Autodesk Inventor part; units mm, degrees
(part 2 of 2)
sketch "Náčrt2 outline for Vysunutí2" plane through (-3.809999, 5.08, 0) normal (0, 1, 0) x (1, 0, 0)
  line L0 (-2.971901, 1.32351) -> (-1.677758, 1.064456)
  line L1 (-2.990322, 1.327194) -> (-2.971901, 1.32351)
  arc A0 (-3.389, 1.845748) -> (-2.990322, 1.327194) centre (-2.881505, 1.82339) ccw
  line L2 (-3.389, 2.240304) -> (-3.389, 1.845748)
  arc A1 (-2.97646, 2.739034) -> (-3.389, 2.240304) centre (-2.881172, 2.240226) ccw
  line L3 (-1.678461, 2.998415) -> (-2.97646, 2.739034)
  arc A2 (-1.27, 3.497336) -> (-1.678461, 2.998415) centre (-1.778009, 3.496575) cw
  line L4 (-1.27, 0.566986) -> (-1.27, 3.497336)
  arc A3 (-1.677758, 1.064456) -> (-1.27, 0.566986) centre (-1.777338, 0.566986) cw
  line L5 (-2.971901, 87.172837) -> (-1.677758, 86.913783)
  line L6 (-2.990322, 87.176521) -> (-2.971901, 87.172837)
  arc A4 (-3.389, 87.695075) -> (-2.990322, 87.176521) centre (-2.881505, 87.672717) ccw
  line L7 (-3.389, 88.089631) -> (-3.389, 87.695075)
  arc A5 (-2.97646, 88.588361) -> (-3.389, 88.089631) centre (-2.881172, 88.089553) ccw
  line L8 (-1.678461, 88.847742) -> (-2.97646, 88.588361)
  arc A6 (-1.27, 89.346664) -> (-1.678461, 88.847742) centre (-1.778009, 89.345902) cw
  line L9 (-1.27, 86.416314) -> (-1.27, 89.346664)
  arc A7 (-1.677758, 86.913783) -> (-1.27, 86.416314) centre (-1.777338, 86.416314) cw
  line L10 (-2.971901, 83.87094) -> (-1.677758, 83.611886)
  line L11 (-2.990322, 83.874624) -> (-2.971901, 83.87094)
  arc A8 (-3.389, 84.393178) -> (-2.990322, 83.874624) centre (-2.881505, 84.37082) ccw
  line L12 (-3.389, 84.78802) -> (-3.389, 84.393178)
  arc A9 (-2.97646, 85.286464) -> (-3.389, 84.78802) centre (-2.881172, 84.787656) ccw
  line L13 (-1.678461, 85.545844) -> (-2.97646, 85.286464)
  arc A10 (-1.27, 86.044766) -> (-1.678461, 85.545844) centre (-1.778009, 86.044005) cw
  line L14 (-1.27, 83.114416) -> (-1.27, 86.044766)
  arc A11 (-1.677758, 83.611886) -> (-1.27, 83.114416) centre (-1.777338, 83.114416) cw
  line L15 (-2.971901, 80.569043) -> (-1.677758, 80.309989)
  line L16 (-2.990322, 80.572727) -> (-2.971901, 80.569043)
  arc A12 (-3.389, 81.091281) -> (-2.990322, 80.572727) centre (-2.881505, 81.068923) ccw
  line L17 (-3.389, 81.486123) -> (-3.389, 81.091281)
  arc A13 (-2.97646, 81.984567) -> (-3.389, 81.486123) centre (-2.881172, 81.485759) ccw
  line L18 (-1.678461, 82.243947) -> (-2.97646, 81.984567)
  arc A14 (-1.27, 82.742869) -> (-1.678461, 82.243947) centre (-1.778009, 82.742108) cw
  line L19 (-1.27, 79.812519) -> (-1.27, 82.742869)
  arc A15 (-1.677758, 80.309989) -> (-1.27, 79.812519) centre (-1.777338, 79.812519) cw
  line L20 (-2.971901, 77.267146) -> (-1.677758, 77.008092)
  line L21 (-2.990322, 77.27083) -> (-2.971901, 77.267146)
  arc A16 (-3.389, 77.789383) -> (-2.990322, 77.27083) centre (-2.881505, 77.767025) ccw
  line L22 (-3.389, 78.184226) -> (-3.389, 77.789383)
  arc A17 (-2.97646, 78.68267) -> (-3.389, 78.184226) centre (-2.881172, 78.183862) ccw
  line L23 (-1.678461, 78.94205) -> (-2.97646, 78.68267)
  arc A18 (-1.27, 79.440972) -> (-1.678461, 78.94205) centre (-1.778009, 79.440211) cw
  line L24 (-1.27, 76.510622) -> (-1.27, 79.440972)
  arc A19 (-1.677758, 77.008092) -> (-1.27, 76.510622) centre (-1.777338, 76.510622) cw
  line L25 (-2.971901, 73.965248) -> (-1.677758, 73.706195)
  line L26 (-2.990322, 73.968933) -> (-2.971901, 73.965248)
  arc A20 (-3.389, 74.487486) -> (-2.990322, 73.968933) centre (-2.881505, 74.465128) ccw
  line L27 (-3.389, 74.882329) -> (-3.389, 74.487486)
  arc A21 (-2.97646, 75.380772) -> (-3.389, 74.882329) centre (-2.881172, 74.881964) ccw
  line L28 (-1.678461, 75.640153) -> (-2.97646, 75.380772)
  arc A22 (-1.27, 76.139075) -> (-1.678461, 75.640153) centre (-1.778009, 76.138314) cw
  line L29 (-1.27, 73.208725) -> (-1.27, 76.139075)
  arc A23 (-1.677758, 73.706195) -> (-1.27, 73.208725) centre (-1.777338, 73.208725) cw
  line L30 (-2.971901, 70.663351) -> (-1.677758, 70.404297)
  line L31 (-2.990322, 70.667035) -> (-2.971901, 70.663351)
  arc A24 (-3.389, 71.185589) -> (-2.990322, 70.667035) centre (-2.881505, 71.163231) ccw
  line L32 (-3.389, 71.580145) -> (-3.389, 71.185589)
  arc A25 (-2.97646, 72.078875) -> (-3.389, 71.580145) centre (-2.881172, 71.580067) ccw
  line L33 (-1.678461, 72.338256) -> (-2.97646, 72.078875)
  arc A26 (-1.27, 72.837178) -> (-1.678461, 72.338256) centre (-1.778009, 72.836416) cw
  line L34 (-1.27, 69.906828) -> (-1.27, 72.837178)
  arc A27 (-1.677758, 70.404297) -> (-1.27, 69.906828) centre (-1.777338, 69.906828) cw
  line L35 (-2.971901, 67.361454) -> (-1.677758, 67.1024)
  line L36 (-2.990322, 67.365138) -> (-2.971901, 67.361454)
  arc A28 (-3.389, 67.883692) -> (-2.990322, 67.365138) centre (-2.881505, 67.861334) ccw
  line L37 (-3.389, 68.278534) -> (-3.389, 67.883692)
  arc A29 (-2.97646, 68.776978) -> (-3.389, 68.278534) centre (-2.881172, 68.27817) ccw
  line L38 (-1.678461, 69.036358) -> (-2.97646, 68.776978)
  arc A30 (-1.27, 69.53528) -> (-1.678461, 69.036358) centre (-1.778009, 69.534519) cw
  line L39 (-1.27, 66.60493) -> (-1.27, 69.53528)
  arc A31 (-1.677758, 67.1024) -> (-1.27, 66.60493) centre (-1.777338, 66.60493) cw
  line L40 (-2.971901, 64.059557) -> (-1.677758, 63.800503)
  line L41 (-2.990322, 64.063241) -> (-2.971901, 64.059557)
  arc A32 (-3.389, 64.581795) -> (-2.990322, 64.063241) centre (-2.881505, 64.559437) ccw
  line L42 (-3.389, 64.976351) -> (-3.389, 64.581795)
  arc A33 (-2.97646, 65.475081) -> (-3.389, 64.976351) centre (-2.881172, 64.976273) ccw
  line L43 (-1.678461, 65.734461) -> (-2.97646, 65.475081)
  arc A34 (-1.27, 66.233383) -> (-1.678461, 65.734461) centre (-1.778009, 66.232622) cw
  line L44 (-1.27, 63.303033) -> (-1.27, 66.233383)
  arc A35 (-1.677758, 63.800503) -> (-1.27, 63.303033) centre (-1.777338, 63.303033) cw
  line L45 (-2.971901, 60.75766) -> (-1.677758, 60.498606)
  line L46 (-2.990322, 60.761344) -> (-2.971901, 60.75766)
  arc A36 (-3.389, 61.279897) -> (-2.990322, 60.761344) centre (-2.881505, 61.257539) ccw
  line L47 (-3.389, 61.67474) -> (-3.389, 61.279897)
  arc A37 (-2.97646, 62.173184) -> (-3.389, 61.67474) centre (-2.881172, 61.674376) ccw
  line L48 (-1.678461, 62.432564) -> (-2.97646, 62.173184)
  arc A38 (-1.27, 62.931486) -> (-1.678461, 62.432564) centre (-1.778009, 62.930725) cw
  line L49 (-1.27, 60.001136) -> (-1.27, 62.931486)
  arc A39 (-1.677758, 60.498606) -> (-1.27, 60.001136) centre (-1.777338, 60.001136) cw
  line L50 (-2.971901, 57.455762) -> (-1.677758, 57.196709)
  line L51 (-2.990322, 57.459447) -> (-2.971901, 57.455762)
  arc A40 (-3.389, 57.978) -> (-2.990322, 57.459447) centre (-2.881505, 57.955642) ccw
  line L52 (-3.389, 58.372843) -> (-3.389, 57.978)
  arc A41 (-2.97646, 58.871286) -> (-3.389, 58.372843) centre (-2.881172, 58.372478) ccw
  line L53 (-1.678461, 59.130667) -> (-2.97646, 58.871286)
  arc A42 (-1.27, 59.629589) -> (-1.678461, 59.130667) centre (-1.778009, 59.628828) cw
  line L54 (-1.27, 56.699239) -> (-1.27, 59.629589)
  arc A43 (-1.677758, 57.196709) -> (-1.27, 56.699239) centre (-1.777338, 56.699239) cw
  line L55 (-2.971901, 54.153865) -> (-1.677758, 53.894811)
  line L56 (-2.990322, 54.15755) -> (-2.971901, 54.153865)
  arc A44 (-3.389, 54.676103) -> (-2.990322, 54.15755) centre (-2.881505, 54.653745) ccw
  line L57 (-3.389, 55.070946) -> (-3.389, 54.676103)
  arc A45 (-2.97646, 55.569389) -> (-3.389, 55.070946) centre (-2.881172, 55.070581) ccw
  line L58 (-1.678461, 55.82877) -> (-2.97646, 55.569389)
  arc A46 (-1.27, 56.327692) -> (-1.678461, 55.82877) centre (-1.778009, 56.32693) cw
  line L59 (-1.27, 53.397342) -> (-1.27, 56.327692)
  arc A47 (-1.677758, 53.894811) -> (-1.27, 53.397342) centre (-1.777338, 53.397342) cw
  line L60 (-2.971901, 50.851968) -> (-1.677758, 50.592914)
  line L61 (-2.990322, 50.855652) -> (-2.971901, 50.851968)
  arc A48 (-3.389, 51.374206) -> (-2.990322, 50.855652) centre (-2.881505, 51.351848) ccw
  line L62 (-3.389, 51.769048) -> (-3.389, 51.374206)
  arc A49 (-2.97646, 52.267492) -> (-3.389, 51.769048) centre (-2.881172, 51.768684) ccw
  line L63 (-1.678461, 52.526873) -> (-2.97646, 52.267492)
  arc A50 (-1.27, 53.025794) -> (-1.678461, 52.526873) centre (-1.778009, 53.025033) cw
  line L64 (-1.27, 50.095444) -> (-1.27, 53.025794)
  arc A51 (-1.677758, 50.592914) -> (-1.27, 50.095444) centre (-1.777338, 50.095444) cw
  line L65 (-2.971901, 47.550071) -> (-1.677758, 47.291017)
  line L66 (-2.990322, 47.553755) -> (-2.971901, 47.550071)
  arc A52 (-3.389, 48.072309) -> (-2.990322, 47.553755) centre (-2.881505, 48.049951) ccw
  line L67 (-3.389, 48.466865) -> (-3.389, 48.072309)
  arc A53 (-2.97646, 48.965595) -> (-3.389, 48.466865) centre (-2.881172, 48.466787) ccw
  line L68 (-1.678461, 49.224975) -> (-2.97646, 48.965595)
  arc A54 (-1.27, 49.723897) -> (-1.678461, 49.224975) centre (-1.778009, 49.723136) cw
  line L69 (-1.27, 46.793547) -> (-1.27, 49.723897)
  arc A55 (-1.677758, 47.291017) -> (-1.27, 46.793547) centre (-1.777338, 46.793547) cw
  line L70 (-2.971901, 44.248174) -> (-1.677758, 43.98912)
  line L71 (-2.990322, 44.251858) -> (-2.971901, 44.248174)
  arc A56 (-3.389, 44.770411) -> (-2.990322, 44.251858) centre (-2.881505, 44.748053) ccw
  line L72 (-3.389, 45.165254) -> (-3.389, 44.770411)
  arc A57 (-2.97646, 45.663698) -> (-3.389, 45.165254) centre (-2.881172, 45.16489) ccw
  line L73 (-1.678461, 45.923078) -> (-2.97646, 45.663698)
  arc A58 (-1.27, 46.422) -> (-1.678461, 45.923078) centre (-1.778009, 46.421239) cw
  line L74 (-1.27, 43.49165) -> (-1.27, 46.422)
  arc A59 (-1.677758, 43.98912) -> (-1.27, 43.49165) centre (-1.777338, 43.49165) cw
  line L75 (-2.971901, 40.946276) -> (-1.677758, 40.687223)
  line L76 (-2.990322, 40.949961) -> (-2.971901, 40.946276)
  arc A60 (-3.389, 41.468514) -> (-2.990322, 40.949961) centre (-2.881505, 41.446156) ccw
  line L77 (-3.389, 41.863071) -> (-3.389, 41.468514)
  arc A61 (-2.97646, 42.3618) -> (-3.389, 41.863071) centre (-2.881172, 41.862993) ccw
  line L78 (-1.678461, 42.621181) -> (-2.97646, 42.3618)
  arc A62 (-1.27, 43.120103) -> (-1.678461, 42.621181) centre (-1.778009, 43.119342) cw
  line L79 (-1.27, 40.189753) -> (-1.27, 43.120103)
  arc A63 (-1.677758, 40.687223) -> (-1.27, 40.189753) centre (-1.777338, 40.189753) cw
  line L80 (-2.971901, 37.644379) -> (-1.677758, 37.385325)
  line L81 (-2.990322, 37.648064) -> (-2.971901, 37.644379)
  arc A64 (-3.389, 38.166617) -> (-2.990322, 37.648064) centre (-2.881505, 38.144259) ccw
  line L82 (-3.389, 38.56146) -> (-3.389, 38.166617)
  arc A65 (-2.97646, 39.059903) -> (-3.389, 38.56146) centre (-2.881172, 38.561095) ccw
  line L83 (-1.678461, 39.319284) -> (-2.97646, 39.059903)
  arc A66 (-1.27, 39.818206) -> (-1.678461, 39.319284) centre (-1.778009, 39.817444) cw
  line L84 (-1.27, 36.887856) -> (-1.27, 39.818206)
  arc A67 (-1.677758, 37.385325) -> (-1.27, 36.887856) centre (-1.777338, 36.887856) cw
  line L85 (-2.971901, 34.342482) -> (-1.677758, 34.083428)
  line L86 (-2.990322, 34.346166) -> (-2.971901, 34.342482)
  arc A68 (-3.389, 34.86472) -> (-2.990322, 34.346166) centre (-2.881505, 34.842362) ccw
  line L87 (-3.389, 35.259562) -> (-3.389, 34.86472)
  arc A69 (-2.97646, 35.758006) -> (-3.389, 35.259562) centre (-2.881172, 35.259198) ccw
  line L88 (-1.678461, 36.017387) -> (-2.97646, 35.758006)
  arc A70 (-1.27, 36.516308) -> (-1.678461, 36.017387) centre (-1.778009, 36.515547) cw
  line L89 (-1.27, 33.585958) -> (-1.27, 36.516308)
  arc A71 (-1.677758, 34.083428) -> (-1.27, 33.585958) centre (-1.777338, 33.585958) cw
  line L90 (-2.971901, 31.040585) -> (-1.677758, 30.781531)
  line L91 (-2.990322, 31.044269) -> (-2.971901, 31.040585)
  arc A72 (-3.389, 31.562823) -> (-2.990322, 31.044269) centre (-2.881505, 31.540465) ccw
  line L92 (-3.389, 31.957665) -> (-3.389, 31.562823)
  arc A73 (-2.97646, 32.456109) -> (-3.389, 31.957665) centre (-2.881172, 31.957301) ccw
  line L93 (-1.678461, 32.715489) -> (-2.97646, 32.456109)
  arc A74 (-1.27, 33.214411) -> (-1.678461, 32.715489) centre (-1.778009, 33.21365) cw
  line L94 (-1.27, 30.284061) -> (-1.27, 33.214411)
  arc A75 (-1.677758, 30.781531) -> (-1.27, 30.284061) centre (-1.777338, 30.284061) cw
  line L95 (-2.971901, 27.738688) -> (-1.677758, 27.479634)
  line L96 (-2.990322, 27.742372) -> (-2.971901, 27.738688)
  arc A76 (-3.389, 28.260925) -> (-2.990322, 27.742372) centre (-2.881505, 28.238567) ccw
  line L97 (-3.389, 28.655768) -> (-3.389, 28.260925)
  arc A77 (-2.97646, 29.154212) -> (-3.389, 28.655768) centre (-2.881172, 28.655404) ccw
  line L98 (-1.678461, 29.413592) -> (-2.97646, 29.154212)
  arc A78 (-1.27, 29.912514) -> (-1.678461, 29.413592) centre (-1.778009, 29.911753) cw
  line L99 (-1.27, 26.982164) -> (-1.27, 29.912514)
  arc A79 (-1.677758, 27.479634) -> (-1.27, 26.982164) centre (-1.777338, 26.982164) cw
  line L100 (-2.971901, 24.436791) -> (-1.677758, 24.177737)
  line L101 (-2.990322, 24.440475) -> (-2.971901, 24.436791)
  arc A80 (-3.389, 24.959028) -> (-2.990322, 24.440475) centre (-2.881505, 24.93667) ccw
  line L102 (-3.389, 25.353585) -> (-3.389, 24.959028)
  arc A81 (-2.97646, 25.852314) -> (-3.389, 25.353585) centre (-2.881172, 25.353507) ccw
  line L103 (-1.678461, 26.111695) -> (-2.97646, 25.852314)
  arc A82 (-1.27, 26.610617) -> (-1.678461, 26.111695) centre (-1.778009, 26.609856) cw
  line L104 (-1.27, 23.680267) -> (-1.27, 26.610617)
  arc A83 (-1.677758, 24.177737) -> (-1.27, 23.680267) centre (-1.777338, 23.680267) cw
  line L105 (-2.971901, 21.134893) -> (-1.677758, 20.875839)
  line L106 (-2.990322, 21.138578) -> (-2.971901, 21.134893)
  arc A84 (-3.389, 21.657131) -> (-2.990322, 21.138578) centre (-2.881505, 21.634773) ccw
  line L107 (-3.389, 22.051688) -> (-3.389, 21.657131)
  arc A85 (-2.97646, 22.550417) -> (-3.389, 22.051688) centre (-2.881172, 22.051609) ccw
  line L108 (-1.678461, 22.809798) -> (-2.97646, 22.550417)
  arc A86 (-1.27, 23.30872) -> (-1.678461, 22.809798) centre (-1.778009, 23.307958) cw
  line L109 (-1.27, 20.37837) -> (-1.27, 23.30872)
  arc A87 (-1.677758, 20.875839) -> (-1.27, 20.37837) centre (-1.777338, 20.37837) cw
  line L110 (-2.971901, 17.832996) -> (-1.677758, 17.573942)
  line L111 (-2.990322, 17.83668) -> (-2.971901, 17.832996)
  arc A88 (-3.389, 18.355234) -> (-2.990322, 17.83668) centre (-2.881505, 18.332876) ccw
  line L112 (-3.389, 18.74979) -> (-3.389, 18.355234)
  arc A89 (-2.97646, 19.24852) -> (-3.389, 18.74979) centre (-2.881172, 18.749712) ccw
  line L113 (-1.678461, 19.507901) -> (-2.97646, 19.24852)
  arc A90 (-1.27, 20.006822) -> (-1.678461, 19.507901) centre (-1.778009, 20.006061) cw
  line L114 (-1.27, 17.076472) -> (-1.27, 20.006822)
  arc A91 (-1.677758, 17.573942) -> (-1.27, 17.076472) centre (-1.777338, 17.076472) cw
  line L115 (-2.971901, 14.531099) -> (-1.677758, 14.272045)
  line L116 (-2.990322, 14.534783) -> (-2.971901, 14.531099)
  arc A92 (-3.389, 15.053337) -> (-2.990322, 14.534783) centre (-2.881505, 15.030979) ccw
  line L117 (-3.389, 15.447893) -> (-3.389, 15.053337)
  arc A93 (-2.97646, 15.946623) -> (-3.389, 15.447893) centre (-2.881172, 15.447815) ccw
  line L118 (-1.678461, 16.206003) -> (-2.97646, 15.946623)
  arc A94 (-1.27, 16.704925) -> (-1.678461, 16.206003) centre (-1.778009, 16.704164) cw
  line L119 (-1.27, 13.774575) -> (-1.27, 16.704925)
  arc A95 (-1.677758, 14.272045) -> (-1.27, 13.774575) centre (-1.777338, 13.774575) cw
  line L120 (-2.971901, 11.229202) -> (-1.677758, 10.970148)
  line L121 (-2.990322, 11.232886) -> (-2.971901, 11.229202)
  arc A96 (-3.389, 11.751439) -> (-2.990322, 11.232886) centre (-2.881505, 11.729081) ccw
  line L122 (-3.389, 12.145996) -> (-3.389, 11.751439)
  arc A97 (-2.97646, 12.644726) -> (-3.389, 12.145996) centre (-2.881172, 12.145918) ccw
  line L123 (-1.678461, 12.904106) -> (-2.97646, 12.644726)
  arc A98 (-1.27, 13.403028) -> (-1.678461, 12.904106) centre (-1.778009, 13.402267) cw
  line L124 (-1.27, 10.472678) -> (-1.27, 13.403028)
  arc A99 (-1.677758, 10.970148) -> (-1.27, 10.472678) centre (-1.777338, 10.472678) cw
  line L125 (-2.971901, 7.927305) -> (-1.677758, 7.668251)
  line L126 (-2.990322, 7.930989) -> (-2.971901, 7.927305)
  arc A100 (-3.389, 8.449542) -> (-2.990322, 7.930989) centre (-2.881505, 8.427184) ccw
  line L127 (-3.389, 8.844099) -> (-3.389, 8.449542)
  arc A101 (-2.97646, 9.342828) -> (-3.389, 8.844099) centre (-2.881172, 8.844021) ccw
  line L128 (-1.678461, 9.602209) -> (-2.97646, 9.342828)
  arc A102 (-1.27, 10.101131) -> (-1.678461, 9.602209) centre (-1.778009, 10.10037) cw
  line L129 (-1.27, 7.170781) -> (-1.27, 10.101131)
  arc A103 (-1.677758, 7.668251) -> (-1.27, 7.170781) centre (-1.777338, 7.170781) cw
  line L130 (-2.971901, 4.625407) -> (-1.677758, 4.366353)
  line L131 (-2.990322, 4.629092) -> (-2.971901, 4.625407)
  arc A104 (-3.389, 5.147645) -> (-2.990322, 4.629092) centre (-2.881505, 5.125287) ccw
  line L132 (-3.389, 5.542202) -> (-3.389, 5.147645)
  arc A105 (-2.97646, 6.040931) -> (-3.389, 5.542202) centre (-2.881172, 5.542123) ccw
  line L133 (-1.678461, 6.300312) -> (-2.97646, 6.040931)
  arc A106 (-1.27, 6.799234) -> (-1.678461, 6.300312) centre (-1.778009, 6.798472) cw
  line L134 (-1.27, 3.868884) -> (-1.27, 6.799234)
  arc A107 (-1.677758, 4.366353) -> (-1.27, 3.868884) centre (-1.777338, 3.868884) cw
  line L135 (-2.971901, 156.512678) -> (-1.677758, 156.253624)
  line L136 (-2.990322, 156.516363) -> (-2.971901, 156.512678)
  arc A108 (-3.389, 157.034916) -> (-2.990322, 156.516363) centre (-2.881505, 157.012558) ccw
  line L137 (-3.389, 157.429759) -> (-3.389, 157.034916)
  arc A109 (-2.97646, 157.928202) -> (-3.389, 157.429759) centre (-2.881172, 157.429394) ccw
  line L138 (-1.678461, 158.187583) -> (-2.97646, 157.928202)
  arc A110 (-1.27, 158.686505) -> (-1.678461, 158.187583) centre (-1.778009, 158.685743) cw
  line L139 (-1.27, 155.756155) -> (-1.27, 158.686505)
  arc A111 (-1.677758, 156.253624) -> (-1.27, 155.756155) centre (-1.777338, 155.756155) cw
  line L140 (-2.971901, 153.210781) -> (-1.677758, 152.951727)
  line L141 (-2.990322, 153.214465) -> (-2.971901, 153.210781)
  arc A112 (-3.389, 153.733019) -> (-2.990322, 153.214465) centre (-2.881505, 153.710661) ccw
  line L142 (-3.389, 154.127862) -> (-3.389, 153.733019)
  arc A113 (-2.97646, 154.626305) -> (-3.389, 154.127862) centre (-2.881172, 154.127497) ccw
  line L143 (-1.678461, 154.885686) -> (-2.97646, 154.626305)
  arc A114 (-1.27, 155.384608) -> (-1.678461, 154.885686) centre (-1.778009, 155.383846) cw
  line L144 (-1.27, 152.454257) -> (-1.27, 155.384608)
  arc A115 (-1.677758, 152.951727) -> (-1.27, 152.454257) centre (-1.777338, 152.454257) cw
  line L145 (-2.971901, 149.908884) -> (-1.677758, 149.64983)
  line L146 (-2.990322, 149.912568) -> (-2.971901, 149.908884)
  arc A116 (-3.389, 150.431122) -> (-2.990322, 149.912568) centre (-2.881505, 150.408764) ccw
  line L147 (-3.389, 150.825964) -> (-3.389, 150.431122)
  arc A117 (-2.97646, 151.324408) -> (-3.389, 150.825964) centre (-2.881172, 150.8256) ccw
  line L148 (-1.678461, 151.583788) -> (-2.97646, 151.324408)
  arc A118 (-1.27, 152.08271) -> (-1.678461, 151.583788) centre (-1.778009, 152.081949) cw
  line L149 (-1.27, 149.15236) -> (-1.27, 152.08271)
  arc A119 (-1.677758, 149.64983) -> (-1.27, 149.15236) centre (-1.777338, 149.15236) cw
  line L150 (-2.971901, 146.606987) -> (-1.677758, 146.347933)
  line L151 (-2.990322, 146.610671) -> (-2.971901, 146.606987)
  arc A120 (-3.389, 147.129224) -> (-2.990322, 146.610671) centre (-2.881505, 147.106866) ccw
  line L152 (-3.389, 147.524067) -> (-3.389, 147.129224)
  arc A121 (-2.97646, 148.022511) -> (-3.389, 147.524067) centre (-2.881172, 147.523703) ccw
  line L153 (-1.678461, 148.281891) -> (-2.97646, 148.022511)
  arc A122 (-1.27, 148.780813) -> (-1.678461, 148.281891) centre (-1.778009, 148.780052) cw
  line L154 (-1.27, 145.850463) -> (-1.27, 148.780813)
  arc A123 (-1.677758, 146.347933) -> (-1.27, 145.850463) centre (-1.777338, 145.850463) cw
  line L155 (-2.971901, 143.30509) -> (-1.677758, 143.046036)
  line L156 (-2.990322, 143.308774) -> (-2.971901, 143.30509)
  arc A124 (-3.389, 143.827327) -> (-2.990322, 143.308774) centre (-2.881505, 143.804969) ccw
  line L157 (-3.389, 144.22217) -> (-3.389, 143.827327)
  arc A125 (-2.97646, 144.720613) -> (-3.389, 144.22217) centre (-2.881172, 144.221805) ccw
  line L158 (-1.678461, 144.979994) -> (-2.97646, 144.720613)
  arc A126 (-1.27, 145.477393) -> (-1.678461, 144.979994) centre (-1.778009, 145.478155) cw
  line L159 (-1.27, 142.548566) -> (-1.27, 145.477393)
  arc A127 (-1.677758, 143.046036) -> (-1.27, 142.548566) centre (-1.777338, 142.548566) cw
  line L160 (-2.971901, 140.003192) -> (-1.677758, 139.744138)
  line L161 (-2.990322, 140.006877) -> (-2.971901, 140.003192)
  arc A128 (-3.389, 140.52543) -> (-2.990322, 140.006877) centre (-2.881505, 140.503072) ccw
  line L162 (-3.389, 140.920273) -> (-3.389, 140.52543)
  arc A129 (-2.97646, 141.418716) -> (-3.389, 140.920273) centre (-2.881172, 140.919908) ccw
  line L163 (-1.678461, 141.678097) -> (-2.97646, 141.418716)
  arc A130 (-1.27, 142.177019) -> (-1.678461, 141.678097) centre (-1.778009, 142.176257) cw
  line L164 (-1.27, 139.246669) -> (-1.27, 142.177019)
  arc A131 (-1.677758, 139.744138) -> (-1.27, 139.246669) centre (-1.777338, 139.246669) cw
  line L165 (-2.971901, 136.701295) -> (-1.677758, 136.442241)
  line L166 (-2.990322, 136.704979) -> (-2.971901, 136.701295)
  arc A132 (-3.389, 137.223533) -> (-2.990322, 136.704979) centre (-2.881505, 137.201175) ccw
  line L167 (-3.389, 137.618376) -> (-3.389, 137.223533)
  arc A133 (-2.97646, 138.116819) -> (-3.389, 137.618376) centre (-2.881172, 137.618011) ccw
  line L168 (-1.678461, 138.3762) -> (-2.97646, 138.116819)
  arc A134 (-1.27, 138.875122) -> (-1.678461, 138.3762) centre (-1.778009, 138.87436) cw
  line L169 (-1.27, 135.944771) -> (-1.27, 138.875122)
  arc A135 (-1.677758, 136.442241) -> (-1.27, 135.944771) centre (-1.777338, 135.944771) cw
  line L170 (-2.971901, 133.399398) -> (-1.677758, 133.140344)
  line L171 (-2.990322, 133.403082) -> (-2.971901, 133.399398)
  arc A136 (-3.389, 133.921636) -> (-2.990322, 133.403082) centre (-2.881505, 133.899278) ccw
  line L172 (-3.389, 134.316478) -> (-3.389, 133.921636)
  arc A137 (-2.97646, 134.814922) -> (-3.389, 134.316478) centre (-2.881172, 134.316114) ccw
  line L173 (-1.678461, 135.074302) -> (-2.97646, 134.814922)
  arc A138 (-1.27, 135.573224) -> (-1.678461, 135.074302) centre (-1.778009, 135.572463) cw
  line L174 (-1.27, 132.642874) -> (-1.27, 135.573224)
  arc A139 (-1.677758, 133.140344) -> (-1.27, 132.642874) centre (-1.777338, 132.642874) cw
  line L175 (-2.971901, 130.097501) -> (-1.677758, 129.838447)
  line L176 (-2.990322, 130.101185) -> (-2.971901, 130.097501)
  arc A140 (-3.389, 130.619739) -> (-2.990322, 130.101185) centre (-2.881505, 130.59738) ccw
  line L177 (-3.389, 131.014581) -> (-3.389, 130.619739)
  arc A141 (-2.97646, 131.513025) -> (-3.389, 131.014581) centre (-2.881172, 131.014217) ccw
  line L178 (-1.678461, 131.772405) -> (-2.97646, 131.513025)
  arc A142 (-1.27, 132.271327) -> (-1.678461, 131.772405) centre (-1.778009, 132.270566) cw
  line L179 (-1.27, 129.340977) -> (-1.27, 132.271327)
  arc A143 (-1.677758, 129.838447) -> (-1.27, 129.340977) centre (-1.777338, 129.340977) cw
  line L180 (-2.971901, 123.493706) -> (-1.677758, 123.234652)
  line L181 (-2.990322, 123.497391) -> (-2.971901, 123.493706)
  arc A144 (-3.389, 124.015944) -> (-2.990322, 123.497391) centre (-2.881505, 123.993586) ccw
  line L182 (-3.389, 124.410787) -> (-3.389, 124.015944)
  arc A145 (-2.97646, 124.90923) -> (-3.389, 124.410787) centre (-2.881172, 124.410422) ccw
  line L183 (-1.678461, 125.168611) -> (-2.97646, 124.90923)
  arc A146 (-1.27, 125.667533) -> (-1.678461, 125.168611) centre (-1.778009, 125.666771) cw
  line L184 (-1.27, 122.737183) -> (-1.27, 125.667533)
  arc A147 (-1.677758, 123.234652) -> (-1.27, 122.737183) centre (-1.777338, 122.737183) cw
  line L185 (-2.971901, 126.795604) -> (-1.677758, 126.53655)
  line L186 (-2.990322, 126.799288) -> (-2.971901, 126.795604)
  arc A148 (-3.389, 127.317841) -> (-2.990322, 126.799288) centre (-2.881505, 127.295483) ccw
  line L187 (-3.389, 127.712684) -> (-3.389, 127.317841)
  arc A149 (-2.97646, 128.211127) -> (-3.389, 127.712684) centre (-2.881172, 127.712319) ccw
  line L188 (-1.678461, 128.470508) -> (-2.97646, 128.211127)
  arc A150 (-1.27, 128.96943) -> (-1.678461, 128.470508) centre (-1.778009, 128.968669) cw
  line L189 (-1.27, 126.03908) -> (-1.27, 128.96943)
  arc A151 (-1.677758, 126.53655) -> (-1.27, 126.03908) centre (-1.777338, 126.03908) cw
  line L190 (-2.971901, 120.191809) -> (-1.677758, 119.932755)
  line L191 (-2.990322, 120.195493) -> (-2.971901, 120.191809)
  arc A152 (-3.389, 120.714047) -> (-2.990322, 120.195493) centre (-2.881505, 120.691689) ccw
  line L192 (-3.389, 121.10889) -> (-3.389, 120.714047)
  arc A153 (-2.97646, 121.607333) -> (-3.389, 121.10889) centre (-2.881172, 121.108525) ccw
  line L193 (-1.678461, 121.866714) -> (-2.97646, 121.607333)
  arc A154 (-1.27, 122.365636) -> (-1.678461, 121.866714) centre (-1.778009, 122.364874) cw
  line L194 (-1.27, 119.435285) -> (-1.27, 122.365636)
  arc A155 (-1.677758, 119.932755) -> (-1.27, 119.435285) centre (-1.777338, 119.435285) cw
  line L195 (-1.678461, 118.564816) -> (-2.97646, 118.305436)
  arc A156 (-1.27, 119.063738) -> (-1.678461, 118.564816) centre (-1.778009, 119.062977) cw
  line L196 (-1.27, 116.133388) -> (-1.27, 119.063738)
  arc A157 (-1.677758, 116.630858) -> (-1.27, 116.133388) centre (-1.777338, 116.133388) cw
  line L197 (-2.971901, 116.889912) -> (-1.677758, 116.630858)
  line L198 (-2.990322, 116.893596) -> (-2.971901, 116.889912)
  arc A158 (-3.389, 117.41215) -> (-2.990322, 116.893596) centre (-2.881505, 117.389792) ccw
  line L199 (-3.389, 117.806706) -> (-3.389, 117.41215)
  arc A159 (-2.97646, 118.305436) -> (-3.389, 117.806706) centre (-2.881172, 117.806628) ccw
  line L200 (-2.971901, 113.588015) -> (-1.677758, 113.328961)
  line L201 (-2.990322, 113.591699) -> (-2.971901, 113.588015)
  arc A160 (-3.389, 114.110253) -> (-2.990322, 113.591699) centre (-2.881505, 114.087895) ccw
  line L202 (-3.389, 114.505095) -> (-3.389, 114.110253)
  arc A161 (-2.97646, 115.003539) -> (-3.389, 114.505095) centre (-2.881172, 114.504731) ccw
  line L203 (-1.678461, 115.262919) -> (-2.97646, 115.003539)
  arc A162 (-1.27, 115.761841) -> (-1.678461, 115.262919) centre (-1.778009, 115.76108) cw
  line L204 (-1.27, 112.831491) -> (-1.27, 115.761841)
  arc A163 (-1.677758, 113.328961) -> (-1.27, 112.831491) centre (-1.777338, 112.831491) cw
  line L205 (-2.971901, 106.98422) -> (-1.677758, 106.725166)
  line L206 (-2.990322, 106.987905) -> (-2.971901, 106.98422)
  arc A164 (-3.389, 107.506458) -> (-2.990322, 106.987905) centre (-2.881505, 107.4841) ccw
  line L207 (-3.389, 107.901301) -> (-3.389, 107.506458)
  arc A165 (-2.97646, 108.399744) -> (-3.389, 107.901301) centre (-2.881172, 107.900936) ccw
  line L208 (-1.678461, 108.659125) -> (-2.97646, 108.399744)
  arc A166 (-1.27, 109.158047) -> (-1.678461, 108.659125) centre (-1.778009, 109.157285) cw
  line L209 (-1.27, 106.227697) -> (-1.27, 109.158047)
  arc A167 (-1.677758, 106.725166) -> (-1.27, 106.227697) centre (-1.777338, 106.227697) cw
  line L210 (-2.971901, 110.286118) -> (-1.677758, 110.027064)
  line L211 (-2.990322, 110.289802) -> (-2.971901, 110.286118)
  arc A168 (-3.389, 110.808355) -> (-2.990322, 110.289802) centre (-2.881505, 110.785997) ccw
  line L212 (-3.389, 111.203198) -> (-3.389, 110.808355)
  arc A169 (-2.97646, 111.701641) -> (-3.389, 111.203198) centre (-2.881172, 111.202834) ccw
  line L213 (-1.678461, 111.961022) -> (-2.97646, 111.701641)
  arc A170 (-1.27, 112.459944) -> (-1.678461, 111.961022) centre (-1.778009, 112.459183) cw
  line L214 (-1.27, 109.529594) -> (-1.27, 112.459944)
  arc A171 (-1.677758, 110.027064) -> (-1.27, 109.529594) centre (-1.777338, 109.529594) cw
  line L215 (-2.971901, 103.682323) -> (-1.677758, 103.423269)
  line L216 (-2.990322, 103.686007) -> (-2.971901, 103.682323)
  arc A172 (-3.389, 104.204561) -> (-2.990322, 103.686007) centre (-2.881505, 104.182203) ccw
  line L217 (-3.389, 104.599404) -> (-3.389, 104.204561)
  arc A173 (-2.97646, 105.097847) -> (-3.389, 104.599404) centre (-2.881172, 104.599039) ccw
  line L218 (-1.678461, 105.357228) -> (-2.97646, 105.097847)
  arc A174 (-1.27, 105.85615) -> (-1.678461, 105.357228) centre (-1.778009, 105.855388) cw
  line L219 (-1.27, 102.925799) -> (-1.27, 105.85615)
  arc A175 (-1.677758, 103.423269) -> (-1.27, 102.925799) centre (-1.777338, 102.925799) cw
  line L220 (-2.971901, 100.380426) -> (-1.677758, 100.121372)
  line L221 (-2.990322, 100.38411) -> (-2.971901, 100.380426)
  arc A176 (-3.389, 100.902664) -> (-2.990322, 100.38411) centre (-2.881505, 100.880306) ccw
  line L222 (-3.389, 101.297506) -> (-3.389, 100.902664)
  arc A177 (-2.97646, 101.79595) -> (-3.389, 101.297506) centre (-2.881172, 101.297142) ccw
  line L223 (-1.678461, 102.05533) -> (-2.97646, 101.79595)
  arc A178 (-1.27, 102.554252) -> (-1.678461, 102.05533) centre (-1.778009, 102.553491) cw
  line L224 (-1.27, 99.623902) -> (-1.27, 102.554252)
  arc A179 (-1.677758, 100.121372) -> (-1.27, 99.623902) centre (-1.777338, 99.623902) cw
  line L225 (-2.971901, 97.078529) -> (-1.677758, 96.819475)
  line L226 (-2.990322, 97.082213) -> (-2.971901, 97.078529)
  arc A180 (-3.389, 97.600767) -> (-2.990322, 97.082213) centre (-2.881505, 97.578409) ccw
  line L227 (-3.389, 97.995609) -> (-3.389, 97.600767)
  arc A181 (-2.97646, 98.494053) -> (-3.389, 97.995609) centre (-2.881172, 97.995245) ccw
  line L228 (-1.678461, 98.753433) -> (-2.97646, 98.494053)
  arc A182 (-1.27, 99.252355) -> (-1.678461, 98.753433) centre (-1.778009, 99.251594) cw
  line L229 (-1.27, 96.322005) -> (-1.27, 99.252355)
  arc A183 (-1.677758, 96.819475) -> (-1.27, 96.322005) centre (-1.777338, 96.322005) cw
  line L230 (-2.971901, 93.776632) -> (-1.677758, 93.517578)
  line L231 (-2.990322, 93.780316) -> (-2.971901, 93.776632)
  arc A184 (-3.389, 94.298869) -> (-2.990322, 93.780316) centre (-2.881505, 94.276511) ccw
  line L232 (-3.389, 94.693712) -> (-3.389, 94.298869)
  arc A185 (-2.97646, 95.192156) -> (-3.389, 94.693712) centre (-2.881172, 94.693348) ccw
  line L233 (-1.678461, 95.451536) -> (-2.97646, 95.192156)
  arc A186 (-1.27, 95.948935) -> (-1.678461, 95.451536) centre (-1.778009, 95.949697) cw
  line L234 (-1.27, 93.020108) -> (-1.27, 95.948935)
  arc A187 (-1.677758, 93.517578) -> (-1.27, 93.020108) centre (-1.777338, 93.020108) cw
  line L235 (-2.971901, 90.474734) -> (-1.677758, 90.215681)
  line L236 (-2.990322, 90.478419) -> (-2.971901, 90.474734)
  arc A188 (-3.389, 90.996972) -> (-2.990322, 90.478419) centre (-2.881505, 90.974614) ccw
  line L237 (-3.389, 91.391815) -> (-3.389, 90.996972)
  arc A189 (-2.97646, 91.890258) -> (-3.389, 91.391815) centre (-2.881172, 91.39145) ccw
  line L238 (-1.678461, 92.149639) -> (-2.97646, 91.890258)
  arc A190 (-1.27, 92.648561) -> (-1.678461, 92.149639) centre (-1.778009, 92.647799) cw
  line L239 (-1.27, 89.718211) -> (-1.27, 92.648561)
  arc A191 (-1.677758, 90.215681) -> (-1.27, 89.718211) centre (-1.777338, 89.718211) cw
extrude "Vysunutí2" add sketch "Náčrt2 outline for Vysunutí2" against normal up to surface (3.81 mm away)
sketch "Náčrt3" plane through (0, 0, 0) normal (0, 0, 1) x (1, 0, 0)
  circle A0 centre (20.1, 3.175) radius 2.25
  line L0 (-31, -3.825) -> (-31, 10.175)
  line L1 (-19, -3.825) -> (-31, -3.825)
  line L2 (-19, -3.825) -> (-19, 10.175)
  line L3 (-31, 10.175) -> (-19, 10.175)
  line L4 (13.6, -3.825) -> (13.6, 10.175)
  line L5 (25.6, -3.825) -> (13.6, -3.825)
  line L6 (25.6, 10.175) -> (25.6, -3.825)
  line L7 (13.6, 10.175) -> (25.6, 10.175)
  line L8 (-19, -3.825) -> (13.6, -3.825)
  circle A1 centre (-25.5, 3.175) radius 2.25
  line L9 (13.6, 10.175) -> (-19, 10.175)
  line L10 (-2.539999, 0) -> (0, 0)
  line L11 (0, 6.35) -> (-2.539999, 6.35)
  point P0 (1.329755, -6.450148)
  point P1 (-31, 3.175)
  point P2 (25.6, 3.175)
  dimension "d12" = 4.5
  dimension "d13" = 5.5
  dimension "d14" = 3.825
  dimension "d15" = 14
  dimension "d16" = 32.6
  dimension "d17" = 12
  dimension "d18" = 12
  dimension "d19" = 5.5
  dimension "d20" = 7
  dimension "d21" = 7
  dimension "d22" = 6.35
  dimension "d23" = 19
  constraints: 20 end point, 2 centre point, 2 midpoint
  measures "d12" diameter of A1
  measures "d13" distance of point (-31, 3.175) A1.centre
  measures "d14" distance from line of L9 L11.start
  measures "d15" distance between parallel lines of L8 L9
  measures "d16" distance between parallel lines of L4 L2
  measures "d17" distance between parallel lines of L2 L0
  measures "d18" distance between parallel lines of L6 L4
  measures "d19" distance of point (25.6, 3.175) A0.centre
  measures "d20" distance from line of L7 A0.centre
  measures "d21" distance from line of L3 A1.centre
  measures "d22" distance between parallel lines of L10 L11
  measures "d23" distance from line of L2 L10.end
extrude "Vysunutí3" [suppressed]
fillet "Zaoblení1" [suppressed]
fillet "Zaoblení2" [suppressed]
sketch "Náčrt4" plane through (0, 0, 4) normal (0, 0, 1) x (1, 0, 0)
  line L0 (25.6, 10.175) -> (-31, 10.175) projected
  line L1 (-31, 10.175) -> (-31, -3.825) projected
  line L2 (-31, -3.825) -> (25.6, -3.825) projected
  line L3 (25.6, -3.825) -> (25.6, 10.175) projected
  circle A0 centre (-25.5, 3.175) radius 2.25 projected
  circle A1 centre (20.1, 3.175) radius 2.25 projected
  point P0 (0, 0)
sketch "Náčrt5" plane through (0, 0, 0) normal (0, 0, 1) x (1, 0, 0)
  line L0 (-2.539999, 6.35) -> (0, 6.35)
  line L1 (0, 6.35) -> (-7.5, 6.35)
  line L2 (-7.5, 6.35) -> (-7.5, 0)
  line L3 (-7.5, 0) -> (0, 0)
  line L4 (0, 0) -> (0, 6.35)
  line L5 (25.6, 10.175) -> (-31, 10.175)
  circle A0 centre (-25.5, 3.175) radius 2.25
  line L6 (-31, 10.175) -> (-31, -3.825)
  circle A1 centre (20.1, 3.175) radius 2.25
  line L7 (-31, -3.825) -> (25.6, -3.825)
  line L8 (25.6, -3.825) -> (25.6, 10.175)
  point P0 (0, 0)
  dimension "d28" = 7.5
  dimension "d29" = 6.35
  constraints: 8 end point, 2 parallel, 1 horizontal, 1 perpendicular
  measures "d28" distance of L0.end L1.end
  measures "d29" distance of L3.end L0.end
extrude "Vysunutí4" add sketch "Náčrt5" along normal blind 4 contours L0 L4 L3 L2 L1
